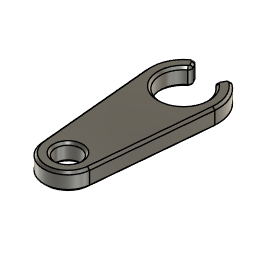
Parametric_PTFE_Umbilcal_guide (Autodesk Fusion 360 archive; units mm, degrees)
design "ptfe_guide"
part number: CableOpeningOnly
Autodesk Fusion 360 part; units mm, degrees
sketch "Sketch1" plane through (0, 0, 0) normal (0, 0, 1) x (1, 0, 0)
  circle A0 centre (0, 0) radius 2.15
  line L0 (0, 0) -> (0, 20) construction
  circle A1 centre (0, 20) radius 4
  circle A2 centre (0, 20) radius 6
  circle A3 centre (0, 0) radius 4.15
  line L1 (5.9743, 19.445) -> (4.1322, -0.3839)
  line L2 (-5.9743, 19.445) -> (-4.1322, -0.3839)
  line L3 (0, 20) -> (0, 26) construction
  line L4 (0, 20) -> (-3, 25.1962)
  line L5 (0, 20) -> (3, 25.1962)
  line L6 (0, 0) -> (0, -4.15) construction
  line L7 (0, 0) -> (-2.075, -3.594)
  line L8 (0, 0) -> (2.075, -3.594)
  dimension "d36" = 4.3
  dimension "d37" = 20
  dimension "d38" = 8
  dimension "d39" = 2
  dimension "d40" = 2
  dimension "d41" = 30
  dimension "d42" = 30
  dimension "d43" = 30
  dimension "d44" = 30
  constraint coincident A0.centre L0.start
  constraint vertical L0
  constraint coincident L0.end A1.centre
  constraint tangent A2 L1
  constraint tangent A3 L1
  constraint tangent A2 L2
  constraint tangent A3 L2
  constraint coincident A2 L3.end
  constraint parallel L0 L3
  constraint coincident A2 L4.end
  constraint coincident A2 L5.end
  constraint coincident A3 L2.end
  constraint coincident A3 L1.end
  constraint coincident A2 L1.start
  constraint coincident A2 L2.start
  constraint coincident A3 L6.end
  constraint parallel L0 L6
  constraint coincident A3 L7.end
  constraint coincident A3 L8.end
  measures "d36" diameter of A0
  measures "d37" distance of A0.centre L0.end
  measures "d38" diameter of A1
  measures "d41" angle of L3 L4
  measures "d42" angle of L3 L5
  measures "d43" angle of L6 L7
  measures "d44" angle of L6 L8
extrude "Extrude6" add sketch "Sketch1" along normal blind 3 contours A0 A3 L7 L8 | A0 A3 L7 L8 | A2 A3 L1 L2 | A1 A2 L4 L5 | A1 A2 L4 L5
extrude "Extrude7" cut sketch "Sketch1" along normal blind 3 contours A1 A2 L4 L5 picked at (-2.3973, 24.7485)
extrude "Extrude8" [suppressed]
fillet "Fillet4" [suppressed]
fillet "Fillet5" radius 0.6 4 edges at (2, 23.4641, 1.5) (3, 25.1962, 1.5) (-3, 25.1962, 1.5) (-2, 23.4641, 1.5)
chamfer "Chamfer4" distance 0.4 angle 45 2 faces at (-4.2595, 12.0282, 3) (-4.2595, 12.0282, 0)
equation "ptfeDiam = 4.3 mm" comment "ptfe Tube diameter or a 2nd cable"
equation "cableDiam = 8 mm" comment "umbilical cable diameter"
equation "offsetCheck = if(offset < 2 mm; 2 mm; offset)"
equation "extrudeThickness = 3 mm" comment "how thick the part is"
equation "ptfeToCable = 20 mm" comment "center to center distance between cable and PTFE tube cant be shorter than the radius of the cable plus the radius of the ptfe tbe, there is a check in place to make sure"
equation "lengthCheck = if(ptfeToCable < ( ( cableDiam / 2 ) + ( 2 * offsetCheck ) + ( ptfeDiam / 2 ) + 0.5 mm ); ( cableDiam / 2 ) + ( 2 * offsetCheck ) + ( ptfeDiam / 2 ) + 0.5 mm; ptfeToCable)"
equation "d36 = ptfeDiam"
equation "d37 = lengthCheck"
equation "d38 = cableDiam"
equation "d39 = offsetCheck"
equation "d40 = offsetCheck"
equation "offset = 2 mm" comment "This is the thickness of the ring around the cable or ptfe tube"
equation "d58 = extrudeThickness"
equation "d60 = extrudeThickness"
equation "d62 = extrudeThickness"
